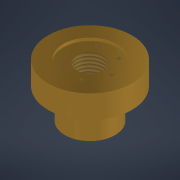
# Autodesk Inventor part: Tuerca
Saved by Autodesk Inventor 2022 (Build 260153000, 153)
## iProperties
Created: 2021-09-10
Part Number: Tuerca
Material: Steel, Mild, Welded
Document SubType Name: Modeling
Designer: Andres
Density: 7.85 g/cm^3
Appearance: Brass - Satin
Author: Andres
Autodesk Inventor part; units mm, degrees
ref_plane "YZ Plane" through (0, 0, 0) normal (1, 0, 0) x (0, 1, 0)
ref_plane "XZ Plane" through (0, 0, 0) normal (0, 1, 0) x (-1, 0, 0)
sketch "Sketch1" plane through (0, 0, 0) normal (0, 1, 0) x (-1, 0, 0)
  circle A0 centre (0, 0) radius 8
  circle A1 centre (0, 0) radius 15
  dimension "d0" = 16
  dimension "d1" = 30
  constraints: 2 centre point, 2 coincident
  measures "d0" diameter of A0
  measures "d1" diameter of A1
extrude "Extrusion1" add sketch "Sketch1" along normal mid plane 30
thread "Thread1" size "TR16x2" class "7H" standard "ISO Metric Trapezoidal Threads" full length
sketch "Sketch2" plane through (0, 15, 0) normal (0, -1, 0) x (1, 0, 0)
  circle A0 centre (0, 0) radius 45
  circle A1 centre (0, 0) radius 15 projected
  circle A2 centre (0, 0) radius 8 projected
  dimension "d6" = 90
  constraints: 1 centre point, 1 coincident
  measures "d6" diameter of A0
extrude "Extrusion2" add sketch "Sketch2" along normal blind 12 contours A0
sketch "Sketch4" plane through (0, 3, 0) normal (0, -1, 0) x (-1, 0, 0)
  circle A0 centre (0, 0) radius 45 projected
  circle A1 centre (0, 0) radius 8 projected
  circle A2 centre (0, 0) radius 15
  circle A3 centre (0, 0) radius 23.5
  dimension "d11" = 30
  dimension "d15" = 47
  constraints: 2 centre point, 2 coincident
  measures "d11" diameter of A2
  measures "d15" diameter of A3
extrude "Extrusion3" cut sketch "Sketch4" against normal blind 3 contours A3
sketch "Sketch6" plane through (0, 15, 0) normal (0, 1, 0) x (1, 0, 0)
  circle A0 centre (0, 0) radius 45 projected
  circle A1 centre (0, 0) radius 8 projected
  circle A2 centre (0, 0) radius 20
  dimension "d27" = 40
  constraints: 1 centre point, 1 coincident
  measures "d27" diameter of A2
ref_plane "Work Plane1" through (-68.5834, 16.8111, -68.5834) normal (0, -1, 0) x (0.8544, 0, 0.5196)
extrude "Extrusion4" add sketch "Sketch6" along normal up to surface (1.8111 mm away) contours A0
body "Solid1"
